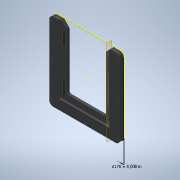
# Autodesk Inventor part: J010353
Saved by Autodesk Inventor 2020.3 (Build 243373000, 373)
## iProperties
RuleStatus: InUse
AfterDocSave0: file://Part Number Cleaner
Created: 2015-02-04
Material: VERO BLACK
Vendor: HHMI: JRC - ID&F
Document SubType Name: Modeling
Designer: NEGRASHOVI
Density: 1.17 g/cm^3
Appearance: Gray
Mass: 200.136 g
Surface Area: 1414.9 cm^2
Volume: 200.136 cm^3
Part Number: J010353
DESIGN DEPARTMENT: HHMI: JRC - ID&F
ALTERED ITEM PART NUMBER: N/A
ALTERED ITEM VENDOR: N/A
ALTERED ITEM DESCRIPTION: N/A
Author: NEGRASHOVI
Revision Number: 0
Autodesk Inventor part; units mm, degrees
ref_plane "XZ Plane" through (0, 0, 0) normal (0, 1, 0) x (-1, 0, 0)
ref_plane "XY Plane" through (0, 0, 0) normal (0, 0, 1) x (1, 0, 0)
sketch "Sketch1" plane through (0, 0, 0) normal (0, 0, 1) x (1, 0, 0)
  line L0 (-50.8, -63.5) -> (50.8, -63.5)
  line L1 (57.15, -57.15) -> (57.15, 57.15)
  line L2 (50.8, 63.5) -> (-50.8, 63.5)
  line L3 (-57.15, 57.15) -> (-57.15, -57.15)
  arc A0 (-50.8, 63.5) -> (-57.15, 57.15) centre (-50.8, 57.15) ccw
  arc A1 (57.15, 57.15) -> (50.8, 63.5) centre (50.8, 57.15) ccw
  arc A2 (50.8, -63.5) -> (57.15, -57.15) centre (50.8, -57.15) ccw
  arc A3 (-57.15, -57.15) -> (-50.8, -63.5) centre (-50.8, -57.15) ccw
  line L4 (-82.8172, 0) -> (87.6474, 0) construction
  line L5 (0, -90.7412) -> (0, 90.7412) construction
  line L6 (-53.975, 57.15) -> (53.975, 57.15) construction
  line L7 (53.975, 57.15) -> (53.975, -60.325) construction
  line L8 (53.975, -60.325) -> (-53.975, -60.325) construction
  line L9 (-53.975, -60.325) -> (-53.975, 57.15) construction
  line L10 (-50.8, 63.5) -> (50.8, 63.5)
  line L11 (50.8, 63.5) -> (50.8, -57.15)
  line L12 (50.8, -57.15) -> (-50.8, -57.15)
  line L13 (-50.8, -57.15) -> (-50.8, 63.5)
  line L14 (-31.75, -38.1) -> (31.75, -38.1)
  line L15 (31.75, -38.1) -> (31.75, 38.1)
  line L16 (31.75, 38.1) -> (-31.75, 38.1)
  line L17 (-31.75, 38.1) -> (-31.75, -38.1)
  circle A4 centre (0, 0) radius 26.67
  line L18 (44.45, 38.1) -> (-44.45, 38.1) construction
  line L19 (-44.45, 38.1) -> (-44.45, -50.8) construction
  line L20 (-44.45, -50.8) -> (44.45, -50.8) construction
  line L21 (44.45, -50.8) -> (44.45, 38.1) construction
  circle A5 centre (44.45, -50.8) radius 2.0955 construction
  circle A6 centre (-44.45, -50.8) radius 2.0955 construction
  circle A7 centre (-44.45, 38.1) radius 2.0955 construction
  circle A8 centre (44.45, 38.1) radius 2.0955 construction
  arc A9 (57.15, -57.15) -> (57.15, -34.6329) centre (49.9095, -45.8915) ccw
  point P0 (0, 63.5)
  point P1 (57.15, 0)
  point P2 (0, 44.45)
  point P3 (0, -60.325)
  point P4 (-40.64, -60.325)
  point P5 (-20.32, -60.325)
  point P6 (20.32, -60.325)
  point P7 (40.64, -60.325)
  point P8 (53.975, 0)
  point P9 (53.975, 34.29)
  point P10 (53.975, -11.43)
  point P11 (53.975, -34.29)
  point P12 (-53.975, 34.29)
  point P13 (-53.975, 0)
  point P14 (-53.975, -11.43)
  point P15 (-53.975, -34.29)
  point P16 (0, 38.1)
  point P17 (31.75, 0)
  point P18 (-53.975, -57.15)
  point P19 (53.975, -57.15)
  point P20 (0, -50.8)
  dimension "d0" = 6.35
  dimension "d1" = 114.3
  dimension "d2" = 127
  dimension "d6" = 19.05
  dimension "d7" = 3.175
  dimension "d8" = 3.175
  dimension "d9" = 6.35
  dimension "d10" = 20.32
  dimension "d11" = 20.32
  dimension "d12" = 22.86
  dimension "d15" = 22.86
  dimension "d16" = 6.35
  dimension "d17" = 6.35
  dimension "d18" = 25.4
  dimension "d19" = 25.4
  dimension "d60" = 22.86
  dimension "d69" = 53.34
  dimension "d86" = 88.9
  dimension "d87" = 4.191
  dimension "d90" = 13.3858
  dimension "d91" = 22.5171
  dimension "d179" = 50.8
  constraints: 40 end point, 19 point on line, 10 centre point, 10 parallel, 10 point on circle, 8 tangent, 7 coincident, 7 symmetric about line, 6 equal radius, 6 midpoint, 6 perpendicular, 5 horizontal, 3 vertical alignment, 2 horizontal alignment, 2 other
  measures "d0" radius of A0
  measures "d1" distance between parallel lines of L1 L3
  measures "d2" distance between parallel lines of L0 L2
  measures "d6" distance from line of point (0, 44.45) L2
  measures "d7" distance between parallel lines of L9 L3
  measures "d8" distance between parallel lines of L8 L0
  measures "d9" distance between parallel lines of L6 L2
  measures "d10" distance of point (-20.32, -60.325) point (0, -60.325)
  measures "d11" distance of point (-40.64, -60.325) point (-20.32, -60.325)
  measures "d12" distance of point (-53.975, 34.29) L6.start
  measures "d15" distance of point (-53.975, -34.29) point (-53.975, -11.43)
  measures "d16" distance between parallel lines of L11 L1
  measures "d17" distance between parallel lines of L0 L12
  measures "d18" distance between parallel lines of L14 L0
  measures "d19" distance between parallel lines of L1 L15
  measures "d60" distance of point (-53.975, -57.15) point (-53.975, -34.29)
  measures "d69" diameter of A4
  measures "d86" distance of L18.start L18.end
  measures "d87" diameter of A5
  measures "d90" radius of A9
  measures "d91" distance of A9.end L1.start
  measures "d179" distance from line of L20 point (0, 0)
extrude "Extrusion2" add sketch "Sketch1" against normal blind 7.1882 contours A3 L3 A0 L13 L12 L11 A1 L1 A2 L0 | L2 L11 L12 L13
sketch "Sketch20" plane through (0, 0, -7.1882) normal (0, 0, -1) x (-1, 0, 0)
  line L0 (-57.15, 57.15) -> (-57.15, -57.15) projected
  arc A0 (-57.15, -57.15) -> (-50.8, -63.5) centre (-50.8, -57.15) ccw projected
  line L1 (-50.8, -63.5) -> (50.8, -63.5) projected
  arc A1 (50.8, -63.5) -> (57.15, -57.15) centre (50.8, -57.15) ccw projected
  line L2 (57.15, -57.15) -> (57.15, 57.15) projected
  arc A2 (57.15, 57.15) -> (50.8, 63.5) centre (50.8, 57.15) ccw projected
  line L3 (50.8, 63.5) -> (-50.8, 63.5) projected
  arc A3 (-50.8, 63.5) -> (-57.15, 57.15) centre (-50.8, 57.15) ccw projected
  line L4 (-56.9468, -57.15) -> (-56.9468, 57.15)
  arc A4 (-50.8, 63.2968) -> (-56.9468, 57.15) centre (-50.8, 57.15) ccw
  line L5 (-50.8, 63.2968) -> (50.8, 63.2968)
  arc A5 (56.9468, 57.15) -> (50.8, 63.2968) centre (50.8, 57.15) ccw
  line L6 (56.9468, 57.15) -> (56.9468, -57.15)
  arc A6 (50.8, -63.2968) -> (56.9468, -57.15) centre (50.8, -57.15) ccw
  line L7 (50.8, -63.2968) -> (-50.8, -63.2968)
  arc A7 (-56.9468, -57.15) -> (-50.8, -63.2968) centre (-50.8, -57.15) ccw
  point P0 (0, 0)
  dimension "d176" = 0.2032
  constraints: 8 end point, 8 point on circle, 4 centre point, 7 other
  measures "d176" distance between parallel lines of L4 L0
extrude "Extrusion17" cut sketch "Sketch20" against normal through all
sketch "Sketch2" plane through (0, 0, -7.1882) normal (0, 0, -1) x (-1, 0, 0)
  point P0 (0, 0)
  point P1 (53.975, 57.15)
  point P2 (53.975, 34.29)
  point P3 (53.975, 0)
  point P4 (53.975, -11.43)
  point P5 (53.975, -34.29)
  point P6 (40.64, -60.325)
  point P7 (20.32, -60.325)
  point P8 (0, -60.325)
  point P9 (-20.32, -60.325)
  point P10 (-40.64, -60.325)
  point P11 (-53.975, -34.29)
  point P12 (-53.975, -11.43)
  point P13 (-53.975, 0)
  point P14 (-53.975, 34.29)
  point P15 (-53.975, 57.15)
  point P16 (-53.975, -57.15)
  point P17 (53.975, -57.15)
hole "Hole2" at (53.975, 57.15, -7.1882) at (53.975, 0, -7.1882) at (0, -60.325, -7.1882) at (-53.975, 0, -7.1882) at (-53.975, 57.15, -7.1882) at (-53.975, -57.15, -7.1882) at (53.975, -57.15, -7.1882) direction (0, 0, 1) diameter 3.2766 end through all countersink diameter 5.715 countersink angle 82 clearance for "Flat Head Machine Screw (82)" size "#4" standard "Ansi Unified Screw Threads"
fillet "Fillet6" radius 3.175 2 edges at (31.75, -38.1, -3.5941) (-31.75, -38.1, -3.5941)
sketch "Sketch63" plane through (0, 0, -7.1882) normal (0, 0, -1) x (-1, 0, 0)
  circle A0 centre (53.975, -57.15) radius 2.8575 projected
  circle A1 centre (53.975, 0) radius 2.8575 projected
  circle A2 centre (-53.975, 0) radius 2.8575 projected
  circle A3 centre (-53.975, 57.15) radius 2.8575 projected
  circle A4 centre (0, -60.325) radius 2.8575 projected
  circle A5 centre (53.975, 57.15) radius 2.8575 projected
  circle A6 centre (-53.975, -57.15) radius 2.8575 projected
  arc A7 (-56.9468, -57.15) -> (-50.8, -63.2968) centre (-50.8, -57.15) ccw projected
  line L0 (-50.8, -63.2968) -> (50.8, -63.2968) projected
  arc A8 (50.8, -63.2968) -> (56.9468, -57.15) centre (50.8, -57.15) ccw projected
  line L1 (56.9468, -57.15) -> (56.9468, 57.15) projected
  arc A9 (56.9468, 57.15) -> (50.8, 63.2968) centre (50.8, 57.15) ccw projected
  line L2 (50.8, 63.2968) -> (-50.8, 63.2968) projected
  arc A10 (-50.8, 63.2968) -> (-56.9468, 57.15) centre (-50.8, 57.15) ccw projected
  line L3 (-56.9468, 57.15) -> (-56.9468, -57.15) projected
  line L4 (-31.75, -34.925) -> (-31.75, 38.1) projected
  line L5 (-31.75, 38.1) -> (31.75, 38.1) projected
  line L6 (31.75, 38.1) -> (31.75, -34.925) projected
  arc A11 (28.575, -38.1) -> (31.75, -34.925) centre (28.575, -34.925) ccw projected
  line L7 (28.575, -38.1) -> (-28.575, -38.1) projected
  arc A12 (-31.75, -34.925) -> (-28.575, -38.1) centre (-28.575, -34.925) ccw projected
  line L8 (-31.75, 38.1) -> (31.75, 38.1)
  line L9 (31.75, 38.1) -> (31.75, 63.2968)
  line L10 (31.75, 63.2968) -> (-31.75, 63.2968)
  line L11 (-31.75, 63.2968) -> (-31.75, 38.1)
  point P0 (0, 0)
  point P1 (-31.75, 63.2968)
  constraints: 8 end point, 3 coincident, 2 parallel, 1 horizontal, 1 perpendicular, 1 point on line
extrude "Extrusion51" cut sketch "Sketch63" against normal through all contours L2 L9 L5 L11
chamfer "Chamfer6" distance 9.525 angle 45 2 edges at (-31.75, 63.2968, -3.5941) (31.75, 63.2968, -3.5941)
fillet "Fillet70" radius 3.175 4 edges at (41.275, 63.2968, -3.5941) (31.75, 53.7718, -3.5941) (-31.75, 53.7718, -3.5941) (-41.275, 63.2968, -3.5941)
sketch "Sketch64" plane through (0, 0, 0) normal (0, 0, 1) x (1, 0, 0)
  line L0 (-31.75, -34.925) -> (-31.75, 52.4567) projected
  line L1 (31.75, 52.4567) -> (31.75, -34.925) projected
  line L2 (-31.75, -38.1) -> (31.75, -38.1) projected
  line L3 (41.275, 63.2968) -> (-41.275, 63.2968)
  line L4 (-41.275, 63.2968) -> (-41.275, -47.625)
  line L5 (-41.275, -47.625) -> (41.275, -47.625)
  line L6 (41.275, -47.625) -> (41.275, 63.2968)
  line L7 (41.275, 63.2968) -> (-41.275, -47.625) construction
  line L8 (-41.275, 63.2968) -> (41.275, -47.625) construction
  line L9 (50.8, 63.2968) -> (-50.8, 63.2968) projected
  point P0 (0, 0)
  point P1 (0, 0)
  point P2 (0, 7.8359)
  point P3 (0, 7.8359)
  dimension "d517" = 9.525
  dimension "d518" = 82.55
  dimension "d519" = 110.9218
  dimension "d520" = 9.525
  dimension "d521" = 0
  constraints: 12 end point, 3 midpoint, 2 parallel, 1 horizontal, 1 perpendicular, 1 vertical alignment
  measures "d517" distance between parallel lines of L2 L5
  measures "d518" distance of L3.start L3.end
  measures "d519" distance of L3.end L4.end
  measures "d520" distance between parallel lines of L0 L4
  measures "d521" distance between parallel lines of L3 L9
extrude "Extrusion52" cut sketch "Sketch64" against normal blind 3.302
ref_plane "Work Plane15" through (36.5125, 0, 0) normal (1, 0, 0) x (0, 1, 0)
sketch "Sketch65" plane through (36.5125, 0, 0) normal (1, 0, 0) x (0, 1, 0)
  line L0 (-34.925, -3.302) -> (52.4567, -3.302) projected
  line L1 (52.4567, -7.1882) -> (52.4567, -3.302) projected
  line L2 (-34.925, -7.1882) -> (52.4567, -7.1882) projected
  line L3 (-34.925, -3.302) -> (-34.925, -7.1882) projected
  line L4 (-34.925, -3.302) -> (52.4567, -3.302) projected
  line L5 (0, 10.2043) -> (0, -61.2256) projected
  line L6 (-34.925, -7.1882) -> (52.4567, -7.1882) construction
  line L7 (52.1462, -7.1882) -> (48.26, -3.302)
  line L8 (27.94, -3.302) -> (24.0538, -7.1882)
  line L9 (50.8171, -7.1882) -> (46.9309, -3.302)
  line L10 (46.9309, -3.302) -> (48.26, -3.302)
  line L11 (52.1462, -7.1882) -> (50.8171, -7.1882)
  line L12 (27.94, -3.302) -> (29.2691, -3.302)
  line L13 (29.2691, -3.302) -> (25.3829, -7.1882)
  line L14 (25.3829, -7.1882) -> (24.0538, -7.1882)
  line L15 (47.4389, -3.81) -> (28.7611, -3.81)
  arc A0 (28.7611, -3.81) -> (47.4389, -3.81) centre (38.1, 33.1277) ccw
  line L16 (46.9309, -3.302) -> (29.2691, -3.302)
  point P0 (0, 0)
  point P1 (38.1, -3.81)
  dimension "d530" = 135
  dimension "d531" = 135
  dimension "d532" = 20.32
  dimension "d533" = 0.9398
  dimension "d534" = 0.9398
  dimension "d535" = 0.508
  dimension "d536" = 38.1
  dimension "d537" = 38.1
  constraints: 20 end point, 9 point on line, 3 collinear, 2 horizontal, 2 parallel, 2 point on circle, 1 centre point, 1 midpoint, 1 vertical alignment
  measures "d530" angle of L0 L7
  measures "d531" angle of L8 L0
  measures "d532" distance of L8.start L7.end
  measures "d533" distance between parallel lines of L7 L9
  measures "d534" distance between parallel lines of L13 L8
  measures "d535" distance between parallel lines of L15 L0
  measures "d536" radius of A0
  measures "d537" distance from line of L5 A0.centre
extrude "Extrusion53" cut sketch "Sketch65" along normal mid plane 2.54 contours L0 L13 L2 L8 | L0 L9 L15 L13 | L0 L7 L2 L9 | L15 A0
fillet "Fillet71" radius 1.27 2 edges at (36.5125, 47.4389, -3.81) (36.5125, 28.7611, -3.81)
pattern_linear "Rectangular Pattern1" count 2 spacing 69.85 along (0, -1, 0) count 2 spacing 73.025 along (-1, 0, 0) of "Extrusion53", "Fillet71"
chamfer "Chamfer7" distance 0.635 angle 45 8 edges at (-35.2425, -31.75, -3.302) (-37.7825, -31.75, -3.302) (-35.2425, 38.1, -3.302) (-37.7825, 38.1, -3.302) (37.7825, 38.1, -3.302) (35.2425, 38.1, -3.302) (35.2425, -31.75, -3.302) (37.7825, -31.75, -3.302)
equation "\"d11\" = d10"
equation "\"d15\" = d12"
equation "\"d60\" = d12"
